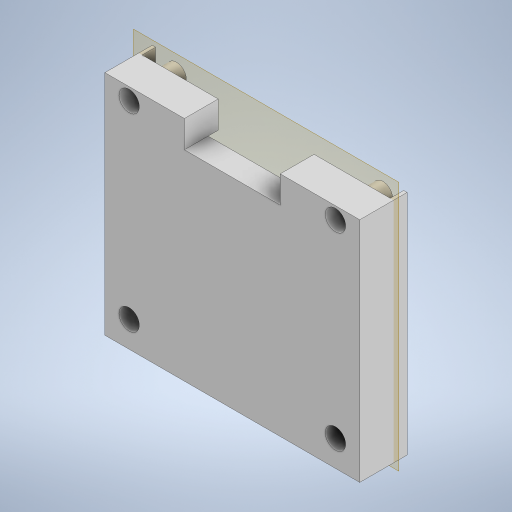
# Autodesk Inventor part: OledCarrier
Saved by Autodesk Inventor 2024.3 (Build 283343000, 343)
## iProperties
Created: 2024-05-11
Part Number: OledCarrier
Material: Generic
Document SubType Name: Modeling
Designer: atrus
Density: 1 g/cm^3
Appearance: Default
Author: atrus
Autodesk Inventor part; units mm, degrees
ref_plane "YZ Plane" through (0, 0, 0) normal (1, 0, 0) x (0, 1, 0)
ref_plane "XZ Plane" through (0, 0, 0) normal (0, 1, 0) x (-1, 0, 0)
ref_plane "XY Plane" through (0, 0, 0) normal (0, 0, 1) x (1, 0, 0)
ref_plane "Work Plane1" through (0, 0, 0) normal (0, 0, 1) x (1, 0, 0)
sketch "Sketch1" plane through (0, 0, 0) normal (0, 0, 1) x (1, 0, 0)
  line L0 (-17.825, 16.8) -> (-17.825, -16.8) construction
  line L1 (-17.825, -16.8) -> (-7, -16.8) construction
  line L2 (-7, -16.8) -> (-7, -13.05) construction
  line L3 (-7, -13.05) -> (7, -13.05) construction
  line L4 (7, -13.05) -> (7, -16.8) construction
  line L5 (7, -16.8) -> (17.825, -16.8) construction
  line L6 (17.825, -16.8) -> (17.825, 16.8) construction
  line L7 (17.825, 16.8) -> (-17.825, 16.8) construction
  circle A0 centre (15.24, 13.97) radius 2.5 construction
  circle A1 centre (-15.24, 13.97) radius 2.5 construction
  circle A2 centre (-15.24, -13.97) radius 2.5 construction
  circle A3 centre (15.24, -13.97) radius 2.5 construction
  line L8 (-18.825, 17.8) -> (-7.08, 17.8)
  line L9 (-7.08, 17.8) -> (-7.08, 11.8)
  line L10 (-7.08, 11.8) -> (7.08, 11.8)
  line L11 (7.08, 11.8) -> (7.08, 17.8)
  line L12 (7.08, 17.8) -> (18.825, 17.8)
  line L13 (18.825, 17.8) -> (18.825, -17.8)
  line L14 (18.825, -17.8) -> (-18.825, -17.8)
  line L15 (-18.825, -17.8) -> (-18.825, 17.8)
  line L16 (-5.08, 14.5) -> (-5.08, 16.3) projected
  line L17 (5.08, 14.5) -> (5.08, 16.3) projected
  point P0 (0, 0)
  dimension "d0" = 1
  dimension "d1" = 1
  dimension "d2" = 1
  dimension "d3" = 1
  dimension "d4" = 2
  dimension "d5" = 5
  constraints: 16 end point, 5 perpendicular, 2 equal length, 1 horizontal, 1 parallel, 1 vertical
  measures "d0" distance between parallel lines of L8 L7
  measures "d1" distance between parallel lines of L0 L15
  measures "d2" distance between parallel lines of L14 L1
  measures "d3" distance between parallel lines of L13 L6
  measures "d4" distance between parallel lines of L9 L16
  measures "d5" distance between parallel lines of L10 L7
extrude "Extrusion1" add sketch "Sketch1" along normal blind 5
sketch "Sketch2" plane through (0, 0, 5) normal (0, 0, 1) x (1, 0, 0)
  circle A0 centre (-15.24, 13.97) radius 1.5 projected
  circle A1 centre (-15.24, -13.97) radius 1.5 projected
  circle A2 centre (15.24, -13.97) radius 1.5 projected
  circle A3 centre (15.24, 13.97) radius 1.5 projected
  point P0 (0, 0)
extrude "Extrusion2" cut sketch "Sketch2" against normal blind 3
sketch "Sketch3" plane through (0, 0, 0) normal (0, 0, -1) x (-1, 0, 0)
  circle A0 centre (-15.24, 13.97) radius 1.5 construction
  circle A1 centre (15.24, 13.97) radius 1.5 construction
  circle A2 centre (15.24, -13.97) radius 1.5 construction
  circle A3 centre (-15.24, -13.97) radius 1.5 construction
  circle A4 centre (-15.24, 13.97) radius 1.45
  circle A5 centre (15.24, 13.97) radius 1.45
  circle A6 centre (15.24, -13.97) radius 1.45
  circle A7 centre (-15.24, -13.97) radius 1.45
  point P0 (0, 0)
  dimension "d10" = 2.9
  constraints: 4 centre point, 4 coincident, 3 equal radius
  measures "d10" diameter of A4
extrude "Extrusion3" add sketch "Sketch3" along normal blind 2 contours A4 | A5
sketch "Sketch4" plane through (0, 0, 0) normal (0, 0, -1) x (-1, 0, 0)
  line L0 (18.825, 17.8) -> (18.825, -17.8) projected
  line L1 (7.08, 17.8) -> (18.825, 17.8) projected
  line L2 (-18.825, 17.8) -> (-7.08, 17.8) projected
  line L3 (-18.825, -17.8) -> (-18.825, 17.8) projected
  line L4 (18.825, -17.8) -> (-18.825, -17.8) projected
  line L5 (7.08, 11.8) -> (7.08, 17.8) projected
  line L6 (7.08, 17.8) -> (7.08, 17.3)
  line L7 (7.08, 17.3) -> (18.325, 17.3)
  line L8 (18.325, 17.3) -> (18.325, -17.3)
  line L9 (18.325, -17.3) -> (-18.325, -17.3)
  line L10 (-18.325, -17.3) -> (-18.325, 17.3)
  line L11 (-18.325, 17.3) -> (-7.08, 17.3)
  line L12 (-7.08, 17.3) -> (-7.08, 17.8)
  line L13 (-18.325, -17.3) -> (-18.325, -17.8)
  line L14 (18.325, -17.3) -> (18.325, -17.8)
  line L15 (18.825, -17.8) -> (-18.825, -17.8) projected
  point P0 (0, 0)
  dimension "d13" = 0.5
  dimension "d14" = 0.5
  dimension "d15" = 0.5
  dimension "d16" = 0.5
  constraints: 18 end point, 6 perpendicular, 3 point on line, 2 parallel, 1 horizontal
  measures "d13" distance between parallel lines of L1 L7
  measures "d14" distance between parallel lines of L4 L9
  measures "d15" distance between parallel lines of L0 L8
  measures "d16" distance between parallel lines of L3 L10
extrude "Extrusion4" add sketch "Sketch4" along normal blind 2 contours L0 L4 L14 L8 L7 L5 L1 | L4 L3 L2 L12 L11 L10 L13
sketch "Sketch5" plane through (7.08, 17.8, 5) normal (0, 1, 0) x (1, 0, 0)
  line L0 (23.7251, 17.6627) -> (-33.6889, 17.6627)
  line L1 (-33.6889, 17.6627) -> (-33.6889, -9.8348)
  line L2 (-33.6889, -9.8348) -> (23.7251, -9.8348)
  line L3 (23.7251, -9.8348) -> (23.7251, 17.6627)
  point P0 (-7.08, 5)
  constraints: 8 end point, 2 parallel, 1 horizontal, 1 perpendicular
extrude "Extrusion5" cut sketch "Sketch5" against normal blind 2
sketch "Sketch6" plane through (0, 0, 0) normal (0, 0, -1) x (-1, 0, 0)
  line L0 (-17.325, 11.8) -> (17.325, 11.8)
  line L1 (17.325, 11.8) -> (17.325, -14.8)
  line L2 (17.325, -14.8) -> (-17.325, -14.8)
  line L3 (-17.325, -14.8) -> (-17.325, 11.8)
  line L4 (-7.08, 11.8) -> (7.08, 11.8) projected
  line L5 (-18.325, -17.8) -> (-18.325, 15.8) projected
  line L6 (18.325, 15.8) -> (18.325, -17.8) projected
  line L7 (18.325, -17.8) -> (-18.325, -17.8) projected
  point P0 (0, 0)
  point P1 (0, 11.8)
  dimension "d21" = 1
  dimension "d22" = 1
  dimension "d23" = 3
  constraints: 8 end point, 2 midpoint, 2 parallel, 1 horizontal, 1 perpendicular
  measures "d21" distance between parallel lines of L5 L3
  measures "d22" distance between parallel lines of L6 L1
  measures "d23" distance between parallel lines of L7 L2
extrude "Extrusion6" cut sketch "Sketch6" against normal blind 1.5
body "Solid1"
